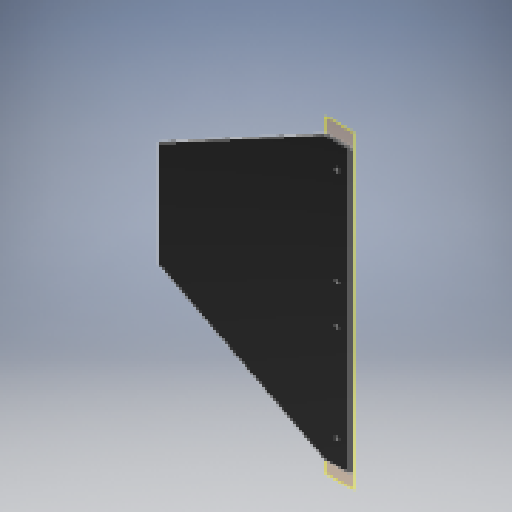
# Autodesk Inventor part: BackPoly
Saved by Autodesk Inventor 2026.1 (Build 301233000, 233)
## iProperties
Created: 2025-09-21
Part Number: BackPoly
Material: Acetal Resin, Black
Document SubType Name: Modeling
Designer: Teddy
Density: 1.425 g/cm^3
Appearance: Smooth - Black
Author: Teddy
Autodesk Inventor part; units mm, degrees
ref_plane "YZ Plane" through (0, 0, 0) normal (1, 0, 0) x (0, 1, 0)
ref_plane "XZ Plane" through (0, 0, 0) normal (0, 1, 0) x (-1, 0, 0)
ref_plane "XY Plane" through (0, 0, 0) normal (0, 0, 1) x (1, 0, 0)
ref_plane "Work Plane1" through (0, 0, 0) normal (0, 0, 1) x (1, 0, 0)
sketch "Sketch1" plane through (0, 0, 0) normal (0, 0, 1) x (1, 0, 0)
  circle A0 centre (0, -152.4) radius 2.1844 projected
  circle A1 centre (0, -25.4) radius 2.1844 projected
  circle A2 centre (0, 25.4) radius 2.1844 projected
  circle A3 centre (0, 152.4) radius 2.1844 projected
  line L0 (-16.6688, -184.15) -> (16.6688, -184.15) projected
  line L1 (16.6687, 184.15) -> (-16.6687, 184.15) projected
  line L2 (16.6688, -184.15) -> (16.6687, 184.15)
  line L3 (-16.6688, -184.15) -> (-84.9313, -127)
  line L4 (-233.7366, -55.6057) -> (-233.7366, -58.7807)
  line L5 (-84.9313, -127) -> (-84.9313, 127)
  line L6 (-84.9313, 127) -> (-16.6687, 184.15)
  point P0 (0, 0)
  dimension "d2" = 254
  dimension "d3" = 101.6
  constraints: 10 end point, 3 vertical, 1 equal length, 2 other
  measures "d2" distance of L3.end L5.end
  measures "d3" distance between parallel lines of L2 L5
extrude "Extrusion1" add sketch "Sketch1" along normal blind 3.175
fillet "Fillet1" radius 12.7 6 edges at (-84.9313, -127, 1.5875) (-16.6688, -184.15, 1.5875) (16.6688, -184.15, 1.5875) (-84.9313, 127, 1.5875) (-16.6687, 184.15, 1.5875) (16.6687, 184.15, 1.5875)
body "Solid1"
